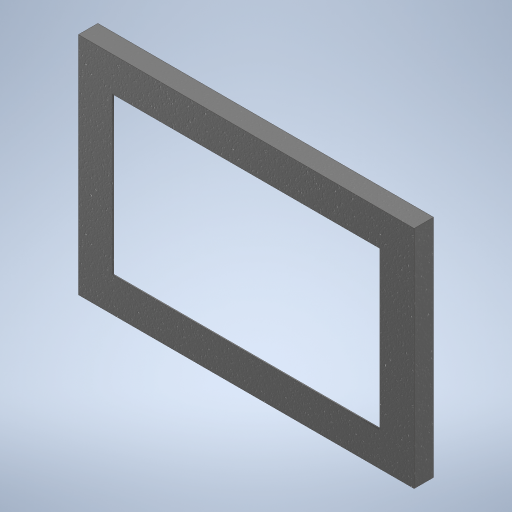
# Autodesk Inventor part: Top Frame Piece
Saved by Autodesk Inventor 2023 (Build 270158000, 158)
## iProperties
Created: 2023-02-23
Part Number: Top Frame Piece
Material: Steel, Mild
Document SubType Name: Modeling
Designer: EvanA
Density: 7.85 g/cm^3
Appearance: Semi-Polished
Author: EvanA
Autodesk Inventor part; units mm, degrees
ref_plane "YZ Plane" through (0, 0, 0) normal (1, 0, 0) x (0, 1, 0)
ref_plane "XZ Plane" through (0, 0, 0) normal (0, 1, 0) x (-1, 0, 0)
ref_plane "XY Plane" through (0, 0, 0) normal (0, 0, 1) x (1, 0, 0)
sketch "Sketch1" plane through (0, 0, 0) normal (0, 0, 1) x (1, 0, 0)
  line L0 (-231.775, 155.575) -> (231.775, 155.575)
  line L1 (231.775, 155.575) -> (231.775, -155.575)
  line L2 (231.775, -155.575) -> (-231.775, -155.575)
  line L3 (-231.775, -155.575) -> (-231.775, 155.575)
  line L4 (-231.775, 155.575) -> (231.775, -155.575) construction
  line L5 (231.775, 155.575) -> (-231.775, -155.575) construction
  line L6 (184.15, -107.95) -> (184.15, 107.95)
  line L7 (184.15, 107.95) -> (-184.15, 107.95)
  line L8 (-184.15, 107.95) -> (-184.15, -107.95)
  line L9 (-184.15, -107.95) -> (184.15, -107.95)
  point P0 (0, 0)
  dimension "d0" = 463.55
  dimension "d1" = 311.15
  dimension "d2" = 47.625
  constraints: 20 end point, 4 parallel, 2 midpoint, 2 perpendicular, 1 horizontal, 3 other
  measures "d0" distance of L1.end L2.end
  measures "d1" distance between parallel lines of L2 L0
  measures "d2" distance between parallel lines of L1 L6
extrude "Extrusion1" add sketch "Sketch1" along normal blind 1.397
sketch "Sketch2" plane through (0, 0, 0) normal (0, 0, -1) x (-1, 0, 0)
  line L0 (-231.775, -155.575) -> (-231.775, 155.575) projected
  line L1 (231.775, -155.575) -> (-231.775, -155.575)
  line L2 (-231.775, -155.575) -> (-231.775, 155.575)
  line L3 (-231.775, 155.575) -> (231.775, 155.575)
  line L4 (231.775, 155.575) -> (231.775, -155.575)
  line L5 (231.775, -155.575) -> (-231.775, 155.575) construction
  line L6 (-231.775, -155.575) -> (231.775, 155.575) construction
  line L7 (230.378, 154.178) -> (-230.378, 154.178)
  line L8 (-230.378, 154.178) -> (-230.378, -154.178)
  line L9 (-230.378, -154.178) -> (230.378, -154.178)
  line L10 (230.378, -154.178) -> (230.378, 154.178)
  point P0 (0, 0)
  dimension "d5" = 1.397
  constraints: 20 end point, 4 parallel, 2 midpoint, 2 perpendicular, 1 horizontal, 3 other
  measures "d5" distance between parallel lines of L3 L7
extrude "Extrusion2" add sketch "Sketch2" along normal blind 25.4
body "Solid1"
